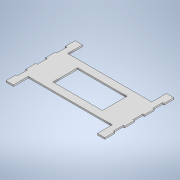
# Autodesk Inventor part: bovenkant
Saved by Autodesk Inventor 2022 (Build 260153000, 153)
## iProperties
Created: 2022-01-28
Part Number: bovenkant
Material: Generic
Document SubType Name: Modeling
Designer: keemi
Density: 1 g/cm^3
Appearance: Default
Author: keemi
Autodesk Inventor part; units mm, degrees
ref_plane "YZ Plane" through (0, 0, 0) normal (1, 0, 0) x (0, 1, 0)
ref_plane "XZ Plane" through (0, 0, 0) normal (0, 1, 0) x (-1, 0, 0)
ref_plane "XY Plane" through (0, 0, 0) normal (0, 0, 1) x (1, 0, 0)
sketch "Sketch1" plane through (0, 0, 0) normal (0, 1, 0) x (-1, 0, 0)
  line L0 (199.9983, 0.0031) -> (184.9983, 0.0007)
  line L1 (199.9983, 0.0031) -> (214.9983, 0.0031) construction
  line L2 (184.9983, 0.0007) -> (184.9983, -29.9993)
  line L3 (184.9983, -29.9993) -> (114.9983, -29.9993)
  line L4 (114.9983, -29.9993) -> (114.9983, 0.0007)
  line L5 (199.9983, -139.9969) -> (184.9983, -139.9969)
  line L6 (199.9983, -139.9969) -> (214.9983, -139.9969) construction
  line L7 (184.9983, -139.9969) -> (184.9983, -109.9969)
  line L8 (184.9983, -109.9969) -> (114.9983, -109.9969)
  line L9 (114.9983, -109.9969) -> (114.9983, -139.9969)
  line L10 (199.9983, 0.0031) -> (196.9983, 0.0026)
  line L11 (196.9983, 0.0026) -> (197.0208, -139.9974)
  line L12 (196.9983, 0.0026) -> (336.9983, 0.0026) construction
  line L13 (199.9983, 0.0031) -> (199.9983, -19.9969)
  line L14 (199.9983, -19.9969) -> (199.9983, -39.9969)
  line L15 (199.9983, -39.9969) -> (199.9983, -59.9969)
  line L16 (199.9983, -59.9969) -> (199.9983, -79.9969)
  line L17 (199.9983, -79.9969) -> (199.9983, -99.9969)
  line L18 (199.9983, -99.9969) -> (199.9983, -119.9969)
  line L19 (199.9983, -119.9969) -> (199.9983, -139.9969)
  line L20 (199.9983, -19.9969) -> (197.0016, -19.9974)
  line L21 (199.9983, -39.9969) -> (197.0048, -39.9974)
  line L22 (199.9983, -59.9969) -> (197.008, -59.9974)
  line L23 (199.9983, -79.9969) -> (197.0112, -79.9974)
  line L24 (199.9983, -99.9969) -> (197.0144, -99.9974)
  line L25 (199.9983, -119.9969) -> (197.0176, -119.9974)
  line L26 (99.9995, -0.013) -> (99.9995, -139.9969)
  line L27 (99.9995, -139.9969) -> (199.9983, -139.9969)
  line L28 (99.9995, -0.013) -> (199.9983, 0.0031)
  line L29 (0.0008, 0.0031) -> (15.0008, 0.0007)
  line L30 (0.0008, 0.0031) -> (-14.9992, 0.0031) construction
  line L31 (15.0008, 0.0007) -> (15.0008, -29.9993)
  line L32 (15.0008, -29.9993) -> (85.0008, -29.9993)
  line L33 (85.0008, -29.9993) -> (85.0008, 0.0007)
  line L34 (85.0008, -109.9969) -> (85.0008, -139.9969)
  line L35 (15.0008, -139.9969) -> (15.0008, -109.9969)
  line L36 (15.0008, -109.9969) -> (85.0008, -109.9969)
  line L37 (0.0008, -139.9969) -> (15.0008, -139.9969)
  line L38 (0.0008, -139.9969) -> (-14.9992, -139.9969) construction
  line L39 (0.0008, 0.0031) -> (3.0008, 0.0026)
  line L40 (3.0008, 0.0026) -> (2.9783, -139.9974)
  line L41 (3.0008, 0.0026) -> (-136.9992, 0.0026) construction
  line L42 (0.0008, 0.0031) -> (0.0008, -19.9969)
  line L43 (0.0008, -19.9969) -> (0.0008, -39.9969)
  line L44 (0.0008, -39.9969) -> (0.0008, -59.9969)
  line L45 (0.0008, -59.9969) -> (0.0008, -79.9969)
  line L46 (0.0008, -79.9969) -> (0.0008, -99.9969)
  line L47 (0.0008, -99.9969) -> (0.0008, -119.9969)
  line L48 (0.0008, -119.9969) -> (0.0008, -139.9969)
  line L49 (0.0008, -19.9969) -> (2.9975, -19.9974)
  line L50 (0.0008, -39.9969) -> (2.9943, -39.9974)
  line L51 (0.0008, -59.9969) -> (2.9911, -59.9974)
  line L52 (0.0008, -79.9969) -> (2.9879, -79.9974)
  line L53 (0.0008, -99.9969) -> (2.9847, -99.9974)
  line L54 (0.0008, -119.9969) -> (2.9815, -119.9974)
  line L55 (99.9995, -139.9969) -> (0.0008, -139.9969)
  line L56 (99.9995, -0.013) -> (0.0008, 0.0031)
  line L57 (114.9983, -109.9969) -> (85.0008, -109.9969)
  line L58 (114.9983, -29.9993) -> (85.0008, -29.9993)
  line L59 (99.9995, -70.0049) -> (99.9995, -95.0049)
  line L60 (99.9995, -95.0049) -> (149.9995, -95.0049)
  line L61 (149.9995, -95.0049) -> (49.9995, -95.0049)
  line L62 (49.9995, -95.0049) -> (49.9995, -45.0049)
  line L63 (49.9995, -45.0049) -> (149.9995, -45.0049)
  line L64 (149.9995, -45.0049) -> (149.9995, -95.0049)
  point P0 (0, 0)
  point P1 (85.0008, -0.0106)
  point P2 (114.9983, -0.0106)
  dimension "d2" = 15
  dimension "d3" = 179.991
  dimension "d4" = 30
  dimension "d5" = 70
  dimension "d6" = 90
  dimension "d12" = 3
  dimension "d13" = 140
  dimension "d14" = 89.991
  dimension "d15" = 20
  dimension "d16" = 20
  dimension "d17" = 20
  dimension "d18" = 20
  dimension "d19" = 20
  dimension "d20" = 20
  dimension "d21" = 20
  dimension "d24" = 25
  dimension "d25" = 50
  dimension "d26" = 100
  dimension "d27" = 50
  constraints: 130 end point, 27 symmetric about line, 23 point on line, 10 perpendicular, 5 horizontal, 3 collinear, 3 parallel, 2 equal length, 2 vertical, 1 midpoint
  measures "d2" distance of L0.start L0.end
  measures "d3" angle of L0 L1
  measures "d4" distance of L0.end L2.end
  measures "d5" distance of L2.end L3.end
  measures "d6" angle of L2 L3
  measures "d12" distance of L0.start L10.end
  measures "d13" distance of L10.end L11.end
  measures "d14" angle of L11 L12
  measures "d15" distance of L0.start L13.end
  measures "d16" distance of L13.end L14.end
  measures "d17" distance of L14.end L15.end
  measures "d18" distance of L15.end L16.end
  measures "d19" distance of L16.end L17.end
  measures "d20" distance of L17.end L18.end
  measures "d21" distance of L18.end L5.start
  measures "d24" distance of L59.start L59.end
  measures "d25" distance of L59.end L60.end
  measures "d26" distance of L62.end L63.end
  measures "d27" distance of L61.end L62.end
extrude "Extrusion1" add sketch "Sketch1" along normal blind 3 contours L13 L20 L11 L0 | L11 L5 L7 L8 L57 L26 L60 L64 L63 L58 L3 L2 L0 | L15 L22 L11 L21 | L17 L24 L11 L23 | L26 L63 L62 L61 L57 L36 L35 L37 L40 L29 L31 L32 L58 | L19 L5 L11 L25 | L40 L49 L42 L29 | L40 L51 L44 L50 | L40 L53 L46 L52 | L37 L48 L54 L40
body "Solid1"
